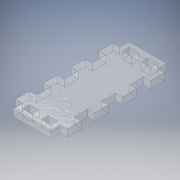
# Autodesk Inventor part: case_side
Saved by Autodesk Inventor 2019 (Build 230136000, 136)
## iProperties
Created: 2019-02-02
Part Number: case_side
Material: Acrylic, Clear
Document SubType Name: Modeling
Designer: suchanek
Density: 1.19 g/cm^3
Appearance: Transparent - Clear
Author: suchanek
Autodesk Inventor part; units mm, degrees
ref_plane "YZ Plane" through (0, 0, 0) normal (1, 0, 0) x (0, 1, 0)
ref_plane "XZ Plane" through (0, 0, 0) normal (0, 1, 0) x (-1, 0, 0)
ref_plane "XY Plane" through (0, 0, 0) normal (0, 0, 1) x (1, 0, 0)
sketch "Sketch1" plane through (0, 0, 0) normal (0, 1, 0) x (-1, 0, 0)
  line L0 (16.25, 50) -> (-16.25, 50)
  line L1 (-16.25, 50) -> (-16.25, -50)
  line L2 (-16.25, -50) -> (16.25, -50)
  line L3 (16.25, -50) -> (16.25, 50)
  line L4 (16.25, 50) -> (-16.25, -50) construction
  line L5 (-16.25, 50) -> (16.25, -50) construction
  line L6 (-12.25, 46) -> (-4, 46)
  line L7 (-4, 46) -> (-4, 40)
  line L8 (-4, 40) -> (-12.25, 40)
  line L9 (-12.25, 40) -> (-12.25, 46)
  line L10 (-16.25, 6) -> (-22.25, 6)
  line L11 (-22.25, 6) -> (-22.25, 18)
  line L12 (-22.25, 18) -> (-16.25, 18)
  line L13 (-16.25, 18) -> (-16.25, 6)
  line L14 (-16.25, 30) -> (-22.25, 30)
  line L15 (-22.25, 30) -> (-22.25, 42)
  line L16 (-22.25, 42) -> (-16.25, 42)
  line L17 (-16.25, 42) -> (-16.25, 30)
  line L18 (0, 0) -> (0, 6.5854)
  line L19 (0, 6.5854) -> (0, 0)
  line L20 (0, 0) -> (-5.5856, 0)
  line L21 (12.25, 46) -> (4, 46)
  line L22 (4, 46) -> (4, 40)
  line L23 (4, 40) -> (12.25, 40)
  line L24 (12.25, 40) -> (12.25, 46)
  line L25 (16.25, 6) -> (22.25, 6)
  line L26 (22.25, 6) -> (22.25, 18)
  line L27 (22.25, 18) -> (16.25, 18)
  line L28 (16.25, 18) -> (16.25, 6)
  line L29 (16.25, 30) -> (22.25, 30)
  line L30 (22.25, 30) -> (22.25, 42)
  line L31 (22.25, 42) -> (16.25, 42)
  line L32 (16.25, 42) -> (16.25, 30)
  line L33 (-12.25, -46) -> (-4, -46)
  line L34 (-4, -46) -> (-4, -40)
  line L35 (-4, -40) -> (-12.25, -40)
  line L36 (-12.25, -40) -> (-12.25, -46)
  line L37 (-16.25, -6) -> (-22.25, -6)
  line L38 (-22.25, -6) -> (-22.25, -18)
  line L39 (-22.25, -18) -> (-16.25, -18)
  line L40 (-16.25, -18) -> (-16.25, -6)
  line L41 (-16.25, -30) -> (-22.25, -30)
  line L42 (-22.25, -30) -> (-22.25, -42)
  line L43 (-22.25, -42) -> (-16.25, -42)
  line L44 (-16.25, -42) -> (-16.25, -30)
  line L45 (4, -40) -> (12.25, -40)
  line L46 (12.25, -46) -> (4, -46)
  line L47 (4, -46) -> (4, -40)
  line L48 (12.25, -40) -> (12.25, -46)
  line L49 (16.25, -18) -> (16.25, -6)
  line L50 (22.25, -42) -> (16.25, -42)
  line L51 (22.25, -30) -> (22.25, -42)
  line L52 (16.25, -6) -> (22.25, -6)
  line L53 (22.25, -6) -> (22.25, -18)
  line L54 (16.25, -42) -> (16.25, -30)
  line L55 (22.25, -18) -> (16.25, -18)
  line L56 (16.25, -30) -> (22.25, -30)
  dimension "d0" = 32.5
  dimension "d1" = 100
  dimension "d2" = 6
  dimension "d3" = 12
  dimension "d4" = 12
  dimension "d5" = 12
  dimension "d6" = 6
  dimension "d7" = 4
  dimension "d8" = 4
  dimension "d9" = 4
  dimension "d10" = 6
  constraints: 114 end point, 36 symmetric about line, 9 equal length, 6 point on line, 5 horizontal, 4 perpendicular, 2 midpoint, 1 vertical
  measures "d0" distance of L0.start L0.end
  measures "d1" distance of L2.end L0.start
  measures "d2" distance between parallel lines of L10 L20
  measures "d3" distance of L10.end L11.end
  measures "d4" distance between parallel lines of L14 L12
  measures "d5" distance of L14.end L15.end
  measures "d6" distance of L10.start L10.end
  measures "d7" distance between parallel lines of L1 L9
  measures "d8" distance between parallel lines of L18 L7
  measures "d9" distance between parallel lines of L0 L6
  measures "d10" distance of L8.end L6.start
extrude "Extrusion1" add sketch "Sketch1" along normal blind 6
body "Solid1"
